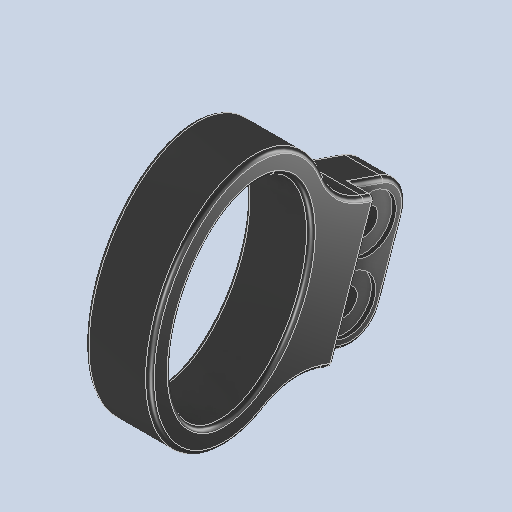
# Autodesk Inventor part: TorsoFrontBumper
Saved by Autodesk Inventor 2024.2 (Build 282272000, 272)
## iProperties
Created: 2024-01-21
Part Number: TorsoFrontBumper
Material: ABS Plastic
Document SubType Name: Modeling
Designer: Masato Kubotera
Density: 1.06 g/cm^3
Appearance: Glossy - Black
Mass: 18.7145 g
Surface Area: 72.9359 cm^2
Volume: 17.6552 cm^3
Catalog Web Link: https://www.poly-maker.jp/polyflex-tpu90.html
Author: Masato Kubotera
Autodesk Inventor part; units mm, degrees
ref_plane "YZ Plane" through (0, 0, 0) normal (1, 0, 0) x (0, 1, 0)
ref_plane "XZ Plane" through (0, 0, 0) normal (0, 1, 0) x (-1, 0, 0)
ref_plane "XY Plane" through (0, 0, 0) normal (0, 0, 1) x (1, 0, 0)
derived "TorsoSideFrame.ipt"
sketch "Sketch5" plane through (0, 0, 0) normal (0, 1, 0) x (-1, 0, 0)
  ellipse E0 centre (-84.0749, 16.6972) end of major axis (-76.7401, 37.9681) minor radius 15 projected
  ellipse E1 centre (-84.0749, 16.6972) end of major axis (-93.0397, -9.3006) minor radius 20 projected
  line L0 (-63.4041, 25.9649) -> (-39.2683, 17.6422) projected
  line L1 (-49.374, -11.6643) -> (-73.5098, -3.3416) projected
  line L2 (-39.2683, 17.6422) -> (-49.374, -11.6643) projected
  line L3 (-48.2759, 36) -> (-65, -12.5) projected
  point P0 (0, 0)
  point P1 (-54.4839, -1.1756)
  point P2 (-49.757, 12.5323)
  point P3 (-63.0819, -6.9375)
  point P4 (-52.9762, 22.3691)
  constraints: 1 other
extrude "Extrusion2" add sketch "Sketch5" against normal blind 10
extrude "Extrusion5" add sketch "Sketch5" along normal blind 5 contours E1 | E1 L0 L3 L1
hole "Hole3" at (54.4839, 0, -1.1756) at (49.757, 0, 12.5323) direction (0, -1, 0) diameter 6 end through all counterbore diameter 12.5 counterbore depth 1
fillet "Fillet9" radius 15 4 edges at (63.4041, -5, 25.9649) (63.4041, 2.5, 25.9649) (73.5098, -5, -3.3416) (73.5098, 2.5, -3.3416)
fillet "Fillet10" radius 1 17 edges at (91.4097, -10, -4.5737) (102.9824, -10, 23.217) (91.4097, 5, -4.5737) (44.3211, -10, 2.989) (57.6584, -10, -8.8076) (47.5527, -10, 20.4989) (52.9762, 2.5, 22.3691) (63.0819, 2.5, -6.9375) (46.1222, 0, 20.0057) (56.2279, 0, -9.3009) (44.3211, 0, 2.989) (54.4066, 5, 22.8624) (102.9824, 5, 23.217) (72.3744, 5, -5.211) (64.5123, 5, -6.4442) (61.3578, 5, 26.7371) (58.029, 5, 7.7158)
fillet "Fillet11" radius 7.5 2 edges at (39.2683, -5, 17.6422) (49.374, -5, -11.6643)
sketch "Sketch1" plane through (0, 0, 0) normal (0, 1, 0) x (-1, 0, 0)
  circle A0 centre (0, 0) radius 18.75 projected
  line L0 (0, 0) -> (0, -161.5) projected
  circle A1 centre (0, 0) radius 29 construction
  line L1 (0, 0) -> (0, 36) projected
  line L2 (0, 36) -> (-48.2759, 36) projected
  line L3 (-65, -12.5) -> (-65, -118) projected
  line L4 (-50, -161.5) -> (-35, -161.5) projected
  line L5 (-35, -161.5) -> (-35, -166.5) projected
  line L6 (-35, -166.5) -> (-10, -166.5) projected
  line L7 (-10, -166.5) -> (-10, -161.5) projected
  line L8 (-10, -161.5) -> (0, -161.5) projected
  line L9 (-60, -40.225) -> (-65, -40.225) projected
  line L10 (-44, -161.5) -> (-44, -155.5) construction
  line L11 (-22.5, -166.5) -> (-22.5, -161.5) construction
  arc A2 (-6, -161.5) -> (-10, -161.5) centre (-8, -161.5) ccw projected
  arc A3 (-35, -161.5) -> (-39, -161.5) centre (-37, -161.5) ccw projected
  line L12 (-65, -12.5) -> (-60, -12.5) construction
  line L13 (-60, -12.5) -> (-60, -106) construction
  line L14 (-62.5, -12.5) -> (-62.5, -106) construction
  line L15 (-65, -40.25) -> (-60, -40.25) construction
  arc A4 (-60, -44.225) -> (-60, -40.225) centre (-60, -42.225) ccw projected
  line L16 (-60, -111) -> (0, -111) construction
  line L17 (-60, -106) -> (0, -106) construction
  line L18 (-60, -108.5) -> (-17.75, -108.5) construction
  line L19 (-9.95, -111.05) -> (-25.55, -111.05) projected
  line L20 (-25.55, -111.05) -> (-25.55, -105.95) projected
  line L21 (-25.55, -105.95) -> (-9.95, -105.95) projected
  line L22 (-9.95, -105.95) -> (-9.95, -111.05) projected
  line L23 (-9.95, -111.05) -> (-25.55, -105.95) construction
  line L24 (-25.55, -111.05) -> (-9.95, -105.95) construction
  line L25 (-25.5, -106) -> (-25.5, -111) construction
  arc A5 (-21.55, -105.95) -> (-25.55, -105.95) centre (-23.55, -105.95) ccw projected
  arc A6 (-25.55, -111.05) -> (-21.55, -111.05) centre (-23.55, -111.05) ccw projected
  line L26 (-22.5, -76.875) -> (-42.5, -76.875) construction
  line L27 (-42.5, -76.875) -> (-42.5, -96.875) construction
  line L28 (-42.5, -96.875) -> (-22.5, -96.875) construction
  line L29 (-22.5, -96.875) -> (-22.5, -76.875) construction
  line L30 (-22.5, -76.875) -> (-42.5, -96.875) construction
  line L31 (-42.5, -76.875) -> (-22.5, -96.875) construction
  line L32 (-45, -74.375) -> (-20, -74.375) construction
  line L33 (-20, -74.375) -> (-20, -99.375) construction
  line L34 (-20, -99.375) -> (-45, -99.375) construction
  line L35 (-45, -99.375) -> (-45, -74.375) construction
  line L36 (-45, -74.375) -> (-20, -99.375) construction
  line L37 (-20, -74.375) -> (-45, -99.375) construction
  line L38 (-50, 31) -> (0, 31) construction
  line L39 (-38.05, 31.05) -> (-14.95, 31.05) projected
  line L40 (-14.95, 31.05) -> (-14.95, 25.95) projected
  line L41 (-14.95, 25.95) -> (-38.05, 25.95) projected
  line L42 (-38.05, 25.95) -> (-38.05, 31.05) projected
  line L43 (-38.05, 31.05) -> (-14.95, 25.95) construction
  line L44 (-14.95, 31.05) -> (-38.05, 25.95) construction
  line L45 (-38.05, 28.5) -> (-14.95, 28.5) construction
  line L46 (-38, 31) -> (-38, 26) construction
  line L47 (-26.5, 31.05) -> (-26.5, 25.95) construction
  line L48 (-15, 31) -> (-15, 26) construction
  arc A7 (-34.05, 31.05) -> (-38.05, 31.05) centre (-36.05, 31.05) ccw projected
  arc A8 (-38.05, 25.95) -> (-34.05, 25.95) centre (-36.05, 25.95) ccw projected
  arc A9 (-14.95, 31.05) -> (-18.95, 31.05) centre (-16.95, 31.05) ccw projected
  arc A10 (-18.95, 25.95) -> (-14.95, 25.95) centre (-16.95, 25.95) ccw projected
  line L49 (-46.4119, -155.5) -> (-3.5, -155.5) projected
  arc A11 (-48.3027, -154.152) -> (-46.4119, -155.5) centre (-46.4119, -153.5) ccw projected
  arc A12 (-3.5, -155.5) -> (-1.5, -153.5) centre (-3.5, -153.5) ccw projected
  circle A13 centre (-41.25, -65.25) radius 2 construction
  line L50 (-3.5, -62.75) -> (-54, -62.75) projected
  line L51 (0, 0) -> (-29, 0) construction
  line L52 (-30.7958, -111) -> (-29.7506, -111) projected
  arc A14 (-27.8427, -112.4) -> (-20.2699, -114.1308) centre (-23.55, -111.05) ccw projected
  line L53 (-1.5, -153.5) -> (-1.5, -113) projected
  arc A15 (-1.5, -113) -> (-3.5, -111) centre (-3.5, -113) ccw projected
  arc A16 (-27.8427, -112.4) -> (-29.7506, -111) centre (-29.7506, -113) ccw projected
  circle A17 centre (-33.5, -108.5) radius 1.75 construction
  arc A18 (-18.8121, -113.5) -> (-20.2699, -114.1308) centre (-18.8121, -115.5) ccw projected
  line L54 (-17.75, -105.95) -> (-17.75, -111.05) construction
  arc A19 (-29.7506, -106) -> (-27.8427, -104.6) centre (-29.7506, -104) ccw projected
  arc A20 (-20.2699, -102.8692) -> (-27.8427, -104.6) centre (-23.55, -105.95) ccw projected
  arc A21 (-20.2699, -102.8692) -> (-18.8121, -103.5) centre (-18.8121, -101.5) ccw projected
  line L55 (-10, -106) -> (-10, -111) construction
  arc A22 (-13.95, -111.05) -> (-9.95, -111.05) centre (-11.95, -111.05) ccw projected
  arc A23 (-5.7494, -111) -> (-7.6573, -112.4) centre (-5.7494, -113) ccw projected
  arc A24 (-15.2301, -114.1308) -> (-16.6879, -113.5) centre (-16.6879, -115.5) ccw projected
  arc A25 (-15.2301, -114.1308) -> (-7.6573, -112.4) centre (-11.95, -111.05) ccw projected
  arc A26 (-9.95, -105.95) -> (-13.95, -105.95) centre (-11.95, -105.95) ccw projected
  arc A27 (-16.6879, -103.5) -> (-15.2301, -102.8692) centre (-16.6879, -101.5) ccw projected
  arc A28 (-7.6573, -104.6) -> (-15.2301, -102.8692) centre (-11.95, -105.95) ccw projected
  arc A29 (-7.6573, -104.6) -> (-5.7494, -106) centre (-5.7494, -104) ccw projected
  line L56 (-18.8121, -103.5) -> (-16.6879, -103.5) projected
  line L57 (-18.8121, -113.5) -> (-16.6879, -113.5) projected
  line L58 (-5.7494, -111) -> (-3.5, -111) projected
  line L59 (-5.7494, -106) -> (-3.5, -106) projected
  arc A30 (-3.5, -106) -> (-1.5, -104) centre (-3.5, -104) ccw projected
  line L60 (-41.25, -65.25) -> (-36.25, -65.25) construction
  line L61 (-60, -44.225) -> (-60, -86.275) projected
  line L62 (-60, -65.25) -> (-65, -65.25) construction
  line L63 (-65, -90.25) -> (-60, -90.25) construction
  arc A31 (-60, -90.275) -> (-60, -86.275) centre (-60, -88.275) ccw projected
  line L64 (-60, -90.275) -> (-65, -90.275) projected
  line L65 (-60, -106) -> (-65, -106) construction
  line L66 (-1.5, -24.2487) -> (-1.5, -60.75) projected
  line L67 (-54, -67.75) -> (-3.5, -67.75) projected
  line L68 (-1.5, -69.75) -> (-1.5, -104) projected
  line L69 (-56, -60.75) -> (-56, -47.5165) projected
  circle A32 centre (-32.5, -86.875) radius 10 projected
  circle A33 centre (-32.5, -86.875) radius 11 projected
  arc A34 (-15.79, 16.0289) -> (-21.7764, 5.6601) centre (0, 0) ccw projected
  arc A35 (-21.7764, -5.6601) -> (-15.79, -16.0289) centre (0, 0) ccw projected
  arc A36 (-5.9864, -21.689) -> (-3.2143, -22.2692) centre (0, 0) ccw projected
  arc A37 (-24.0442, 4.191) -> (-24.0442, -4.191) centre (-24.75, 0) ccw projected
  line L70 (-48.2759, 36) -> (-65, -12.5) projected
  arc A38 (-42.9869, 36) -> (-50, 31) centre (-42.9869, 28.5817) ccw projected
  line L71 (-75.1102, 42.6949) -> (-93.0397, -9.3006) construction
  ellipse E0 centre (-84.0749, 16.6972) end of major axis (-76.7401, 37.9681) minor radius 15 construction
  ellipse E1 centre (-84.0749, 16.6972) end of major axis (-93.0397, -9.3006) minor radius 20 construction
  line L72 (-75.1102, 42.6949) -> (-76.7401, 37.9681) construction
  line L73 (-105, 43.5) -> (-105, 11.4504) construction
  line L74 (-84.0749, 16.6972) -> (-58.029, 7.7158) construction
  line L75 (-63.4041, 25.9649) -> (-39.2683, 17.6422) construction
  line L76 (-39.2683, 17.6422) -> (-49.374, -11.6643) construction
  line L77 (-49.374, -11.6643) -> (-73.5098, -3.3416) construction
  line L78 (-79.9787, 43.5) -> (-105, 43.5) construction
  line L79 (-47.0676, 20.3317) -> (-57.1733, -8.9749) construction
  circle A39 centre (-49.757, 12.5323) radius 6.25 construction
  circle A40 centre (-54.4839, -1.1756) radius 6.25 construction
  line L80 (-1, 13.5) -> (-28, 13.5) construction
  line L81 (-28, 13.5) -> (-28, -13.5) construction
  line L82 (-28, -13.5) -> (-1, -13.5) construction
  line L83 (-1, -13.5) -> (-1, 13.5) construction
  line L84 (-1, 13.5) -> (-28, -13.5) construction
  line L85 (-28, 13.5) -> (-1, -13.5) construction
  line L86 (0, -65.25) -> (-64.9996, -65.25) construction
  line L87 (-50, -161.5) -> (-65, -118) projected
  line L88 (-18.3182, 21.5) -> (-45.3395, 21.5) projected
  arc A41 (-16.4164, 20.1189) -> (-15.6516, 18.7274) centre (-12.375, 21.4341) ccw projected
  arc A42 (-55.5, -46.1936) -> (-58.5, -36.4155) centre (-60, -42.225) ccw projected
  arc A43 (-48.7278, 6.3677) -> (-46.4104, 17.8109) centre (-49.757, 12.5323) ccw projected
  arc A44 (-48.7278, 6.3677) -> (-49.8737, 3.0445) centre (-48.3985, 4.395) ccw projected
  arc A45 (-56.6994, -7.0197) -> (-49.8737, 3.0445) centre (-54.4839, -1.1756) ccw projected
  line L89 (-38, 26) -> (-15, 26) construction
  line L90 (-59.2992, -8.2378) -> (-59.8907, -9.9535) projected
  line L91 (-48.3027, -154.152) -> (-49.1959, -151.5616) projected
  arc A46 (-47.8996, -149) -> (-48.7278, -136.8677) centre (-49.757, -143.0323) ccw projected
  arc A47 (-49.8737, -133.5445) -> (-48.7278, -136.8677) centre (-48.3985, -134.895) ccw projected
  arc A48 (-49.8737, -133.5445) -> (-56.6994, -123.4803) centre (-54.4839, -129.3244) ccw projected
  line L92 (-59.2992, -122.2622) -> (-59.8907, -120.5465) projected
  line L93 (-60, -119.8946) -> (-60, -113) projected
  circle A49 centre (-41.25, -65.25) radius 1 construction
  line L94 (-45, -86.875) -> (-20, -86.875) construction
  arc A50 (-45.3395, 21.5) -> (-46.4104, 17.8109) centre (-45.3395, 19.5) ccw projected
  arc A51 (-56.6994, -7.0197) -> (-59.2992, -8.2378) centre (-57.4084, -8.8898) ccw projected
  arc A52 (-16.4164, 20.1189) -> (-18.3182, 21.5) centre (-18.3182, 19.5) ccw projected
  arc A53 (-15.79, 16.0289) -> (-15.6516, 18.7274) centre (-17.1936, 17.4537) ccw projected
  arc A54 (-24.0442, 4.191) -> (-21.7764, 5.6601) centre (-23.7121, 6.1632) ccw projected
  arc A55 (-21.7764, -5.6601) -> (-24.0442, -4.191) centre (-23.7121, -6.1632) ccw projected
  arc A56 (-15.6516, -18.7274) -> (-15.79, -16.0289) centre (-17.1936, -17.4537) ccw projected
  arc A57 (-5.9864, -21.689) -> (-8.3926, -22.9184) centre (-6.5186, -23.6169) ccw projected
  arc A58 (-60, -34.479) -> (-58.5, -36.4155) centre (-58, -34.479) ccw projected
  line L95 (-40, -42.225) -> (-60, -42.225) construction
  circle A59 centre (-33.5, -108.5) radius 3.25 construction
  arc A60 (-35.174, -111.2857) -> (-31.826, -111.2857) centre (-33.5, -108.5) ccw projected
  line L96 (-36.2042, -111) -> (-58, -111) projected
  line L97 (-36.2042, -106) -> (-58, -106) projected
  arc A61 (-31.826, -105.7143) -> (-35.174, -105.7143) centre (-33.5, -108.5) ccw projected
  line L98 (-30.7958, -106) -> (-29.7506, -106) projected
  arc A62 (-58.5, -94.0845) -> (-55.5, -84.3064) centre (-60, -88.275) ccw projected
  arc A63 (-58.5, -94.0845) -> (-60, -96.021) centre (-58, -96.021) ccw projected
  line L99 (-56, -69.75) -> (-56, -82.9835) projected
  line L100 (-60, -96.021) -> (-60, -104) projected
  arc A64 (-36.2042, -106) -> (-35.174, -105.7143) centre (-36.2042, -104) ccw projected
  arc A65 (-35.174, -111.2857) -> (-36.2042, -111) centre (-36.2042, -113) ccw projected
  arc A66 (-60, -104) -> (-58, -106) centre (-58, -104) ccw projected
  arc A67 (-58, -111) -> (-60, -113) centre (-58, -113) ccw projected
  circle A68 centre (-36.25, -65.25) radius 2 construction
  arc A69 (-31.826, -105.7143) -> (-30.7958, -106) centre (-30.7958, -104) ccw projected
  arc A70 (-30.7958, -111) -> (-31.826, -111.2857) centre (-30.7958, -113) ccw projected
  arc A71 (-47.8996, -149) -> (-49.1959, -151.5616) centre (-47.3052, -150.9096) ccw projected
  arc A72 (-59.2992, -122.2622) -> (-56.6994, -123.4803) centre (-57.4084, -121.6102) ccw projected
  arc A73 (-60, -119.8946) -> (-59.8907, -120.5465) centre (-58, -119.8946) ccw projected
  arc A74 (-60, -119.8946) -> (-59.8907, -120.5465) centre (-58, -119.8946) ccw projected
  arc A75 (-56, -82.9835) -> (-55.5, -84.3064) centre (-54, -82.9835) ccw projected
  arc A76 (-54, -67.75) -> (-56, -69.75) centre (-54, -69.75) ccw projected
  arc A77 (-56, -60.75) -> (-54, -62.75) centre (-54, -60.75) ccw projected
  arc A78 (-55.5, -46.1936) -> (-56, -47.5165) centre (-54, -47.5165) ccw projected
  arc A79 (-1.5, -69.75) -> (-3.5, -67.75) centre (-3.5, -69.75) ccw projected
  arc A80 (-3.5, -62.75) -> (-1.5, -60.75) centre (-3.5, -60.75) ccw projected
  line L101 (-18.3182, -21.5) -> (-58, -21.5) projected
  arc A81 (-18.3182, -21.5) -> (-16.4164, -20.1189) centre (-18.3182, -19.5) ccw projected
  arc A82 (-15.6516, -18.7274) -> (-16.4164, -20.1189) centre (-12.375, -21.4341) ccw projected
  arc A83 (-14.5, -25.1147) -> (-8.3926, -22.9184) centre (-12.375, -21.4341) ccw projected
  line L102 (-16.0857, -24.5) -> (-58, -24.5) projected
  arc A84 (-1.5, -24.2487) -> (-3.2143, -22.2692) centre (-3.5, -24.2487) ccw projected
  line L103 (-60, -10.6054) -> (-60, -19.5) projected
  line L104 (-60, -26.5) -> (-60, -34.479) projected
  arc A85 (-59.8907, -9.9535) -> (-60, -10.6054) centre (-58, -10.6054) ccw projected
  arc A86 (-60, -19.5) -> (-58, -21.5) centre (-58, -19.5) ccw projected
  arc A87 (-58, -24.5) -> (-60, -26.5) centre (-58, -26.5) ccw projected
  arc A88 (-15.0479, -24.7903) -> (-14.5, -25.1147) centre (0, 0) ccw projected
  arc A89 (-15.0479, -24.7903) -> (-16.0857, -24.5) centre (-16.0857, -26.5) ccw projected
  point P0 (-16.05, -9.6933)
  point P1 (-12.375, -21.4341)
  point P2 (12.375, -21.4341)
  point P3 (24.75, 0)
  point P4 (12.375, 21.4341)
  point P5 (-26.5, 28.5)
  point P6 (-60, -106)
  point P7 (-46, 28.5)
  point P8 (-56, -62.75)
  point P9 (-1.5, -155.5)
  point P10 (-5, -161.5)
  point P11 (-28.0497, -111)
  point P12 (-28.0239, -110.5665)
  point P13 (-1.5, -62.75)
  point P14 (-7.4503, -111)
  point P15 (-56, -67.75)
  point P16 (-1.5, -67.75)
  point P17 (-1.5, -22.4499)
  point P18 (-38, 28.5)
  point P19 (-14.5, 0)
  point P20 (-1, 0)
  point P21 (-16.6245, 21.5)
  point P22 (-56, -46.6971)
  point P23 (-60, -36.225)
  point P24 (-49.9833, 18.7782)
  point P25 (-58.5118, -5.9545)
  point P26 (-60, -10.2703)
  point P27 (-46.2796, -23.3529)
  point P28 (-31.2796, -23.3529)
  point P29 (-46.2796, -46.6256)
  point P30 (-62.5, -30.25)
  point P31 (-62.5, -100.25)
  point P32 (-49.9833, -149.2782)
  point P33 (-58.5118, -124.5455)
  point P34 (-60, -120.2297)
  point P35 (-36.05, 23.95)
  point P36 (-31.4233, -111)
  point P37 (-31.4233, -106)
  point P38 (-56, -83.8029)
  point P39 (-40, -88.275)
  point P40 (-15.5161, -24.5)
  constraints: 5 other
body "Solid2"
